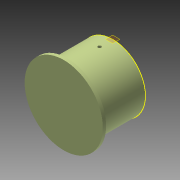
# Autodesk Inventor part: Delvotec-Saughalterung
Saved by Autodesk Inventor 2013 (Build 170138000, 138)
## iProperties
Created: 2014-01-06
Part Number: Delvotec-Saughalterung
Material: Allgemein
Document SubType Name: Modeling
Designer: Frank Meier
Density: 1 g/cm^3
Author: Frank Meier
Autodesk Inventor part; units mm, degrees
ref_plane "YZ Plane" through (0, 0, 0) normal (1, 0, 0) x (0, 1, 0)
ref_plane "XZ Plane" through (0, 0, 0) normal (0, 1, 0) x (-1, 0, 0)
ref_plane "XY Plane" through (0, 0, 0) normal (0, 0, 1) x (1, 0, 0)
sketch "Skizze1" plane through (0, 0, 0) normal (0, 0, 1) x (1, 0, 0)
  line L0 (0, 0) -> (0, 100)
  line L1 (0, 100) -> (-30, 100)
  line L2 (-30, 100) -> (-30, 150)
  line L3 (-30, 150) -> (-100, 150)
  line L4 (-100, 150) -> (-100, 10)
  line L5 (-100, 10) -> (-120, 10)
  line L6 (-120, 10) -> (-120, 0)
  line L7 (-120, 0) -> (0, 0)
  dimension "d0" = 120
  dimension "d2" = 100
  dimension "d3" = 30
  dimension "d4" = 50
  dimension "d5" = 10
  dimension "d6" = 150
  constraints: 16 end point, 6 parallel, 1 perpendicular, 1 vertical
  measures "d0" distance between parallel lines of L0 L6
  measures "d2" distance between parallel lines of L0 L4
  measures "d3" distance between parallel lines of L0 L2
  measures "d4" distance between parallel lines of L1 L3
  measures "d5" distance between parallel lines of L7 L5
  measures "d6" distance between parallel lines of L7 L3
revolve "Umdrehung1" add sketch "Skizze1" angle 360 about axis through (0, 0, 0) along (0, 1, 0)
sketch "Skizze2" plane through (0, 150, 0) normal (0, 1, 0) x (1, 0, 0)
  circle A0 centre (0, 0) radius 100 projected
  line L0 (70, -60) -> (-70, -60)
  line L1 (-70, -60) -> (-70, 60)
  line L2 (-70, 60) -> (70, 60)
  line L3 (70, 60) -> (70, -60)
  line L4 (70, -60) -> (-70, 60) construction
  line L5 (-70, -60) -> (70, 60) construction
  point P0 (-60, 63.5)
  point P1 (60, 63.5)
  point P2 (73.5, 50)
  point P3 (73.5, -50)
  point P4 (60, -63.5)
  point P5 (-60, -63.5)
  point P6 (-73.5, -50)
  point P7 (-73.5, 50)
  dimension "d8" = 140
  dimension "d10" = 120
  dimension "d11" = 10
  dimension "d12" = 3.5
  dimension "d13" = 10
  dimension "d14" = 3.5
  dimension "d16" = 3.5
  dimension "d17" = 3.5
  dimension "d18" = 3.5
  dimension "d19" = 3.5
  dimension "d20" = 3.5
  dimension "d21" = 3.5
  dimension "d22" = 10
  dimension "d23" = 10
  dimension "d24" = 10
  dimension "d25" = 10
  dimension "d26" = 10
  dimension "d27" = 10
  constraints: 12 end point, 2 midpoint, 2 parallel, 1 horizontal, 1 perpendicular
  measures "d8" distance between parallel lines of L3 L1
  measures "d10" distance between parallel lines of L0 L2
  measures "d11" distance from line of L1 point (-60, 63.5)
  measures "d12" distance from line of L2 point (-60, 63.5)
  measures "d13" distance from line of L3 point (60, 63.5)
  measures "d14" distance from line of L2 point (60, 63.5)
  measures "d16" distance from line of L3 point (73.5, -50)
  measures "d17" distance from line of point (73.5, 50) L3
  measures "d18" distance from line of L0 point (60, -63.5)
  measures "d19" distance from line of L0 point (-60, -63.5)
  measures "d20" distance from line of L1 point (-73.5, -50)
  measures "d21" distance from line of L1 point (-73.5, 50)
  measures "d22" distance from line of L2 point (-73.5, 50)
  measures "d23" distance from line of L0 point (-73.5, -50)
  measures "d24" distance from line of L1 point (-60, -63.5)
  measures "d25" distance from line of L3 point (60, -63.5)
  measures "d26" distance from line of point (73.5, -50) L0
  measures "d27" distance from line of L2 point (73.5, 50)
hole "Bohrung1" at (-60, 150, -63.5) at (60, 150, -63.5) at (73.5, 150, -50) at (73.5, 150, 50) at (60, 150, 63.5) at (-60, 150, 63.5) at (-73.5, 150, 50) at (-73.5, 150, -50) direction (0, -1, 0) diameter 3.242 depth 12 tip angle 118 thread size "M4x0.7" class "6H" standard "ISO Metric profile"
sketch "Skizze3" plane through (0, 150, 0) normal (0, 1, 0) x (1, 0, 0)
  circle A0 centre (-73.5, -50) radius 1.621 projected
  circle A1 centre (60, -63.5) radius 1.621 projected
  circle A2 centre (73.5, 50) radius 1.621 projected
  circle A3 centre (-60, 63.5) radius 1.621 projected
  circle A4 centre (60, 63.5) radius 1.621 projected
  circle A5 centre (73.5, -50) radius 1.621 projected
  circle A6 centre (-60, -63.5) radius 1.621 projected
  circle A7 centre (-73.5, 50) radius 1.621 projected
  circle A8 centre (0, 0) radius 30 projected
  circle A9 centre (0, 0) radius 100 projected
  line L0 (0, 0) -> (0, -100)
  constraints: 2 end point, 1 vertical, 1 vertical alignment, 1 other
ref_plane "Arbeitsebene1" through (0, 150, 100) normal (0, 0, 1) x (1, 0, 0)
sketch "Skizze4" plane through (0, 150, 100) normal (0, 0, 1) x (1, 0, 0)
  line L0 (100, 0) -> (-100, 0) projected
  point P0 (0, -150)
  point P1 (0, -40)
  dimension "d35" = 40
  dimension "d36" = 100
  measures "d35" distance from line of L0 point (0, -40)
  measures "d36" horizontal distance of L0.end point (0, -40)
hole "Bohrung2" at (0, 110, 100) direction (0, 0, -1) diameter 10 depth 100 tip angle 118
